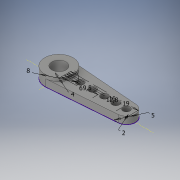
# Autodesk Inventor part: Servo-Arm-20mm
Saved by Autodesk Inventor 2018.2 (Build 222227000, 227)
## iProperties
Created: 2018-02-17
Part Number: Servo-Arm-20mm
Material: Generisch
Document SubType Name: Modeling
Designer: JochenAlt
Density: 1 g/cm^3
Appearance: Vorgabe
Author: JochenAlt
Autodesk Inventor part; units mm, degrees
ref_plane "YZ Plane" through (0, 0, 0) normal (1, 0, 0) x (0, 1, 0)
ref_plane "XZ Plane" through (0, 0, 0) normal (0, 1, 0) x (-1, 0, 0)
ref_plane "XY Plane" through (0, 0, 0) normal (0, 0, 1) x (1, 0, 0)
sketch "Skizze1" plane through (0, 0, 0) normal (0, 0, 1) x (1, 0, 0)
  line L0 (0, 5.6) -> (0, -5.6) construction
  line L1 (-9.1, 0) -> (26.6, 0) construction
  circle A0 centre (0, 0) radius 2
  circle A1 centre (9.5, 0) radius 1
  circle A2 centre (16, 0) radius 1
  circle A3 centre (19, 0) radius 1
  arc A4 (19.1974, -2.4922) -> (19.1974, 2.4922) centre (19, 0) ccw
  arc A5 (0.3158, 3.9875) -> (0.3158, -3.9875) centre (0, 0) ccw
  line L2 (0.3158, 3.9875) -> (19.1974, 2.4922)
  line L3 (0.3158, -3.9875) -> (19.1974, -2.4922)
  circle A6 centre (6, 0) radius 1
  circle A7 centre (12.8, 0) radius 1
  circle A8 centre (0, 0) radius 4
  point P0 (0.5263, 3.9652)
  point P1 (0.6579, -1.8887)
  point P2 (0.6579, 1.8887)
  dimension "d0" = 9.5
  dimension "d1" = 16
  dimension "d2" = 19
  dimension "d3" = 5
  dimension "d4" = 2
  dimension "d5" = 4
  dimension "d6" = 8
  dimension "d16" = 6
  dimension "d17" = 12.8
  constraints: 8 centre point, 7 point on circle, 5 point on line, 4 coincident, 4 end point, 4 equal radius, 4 tangent, 3 other
  measures "d0" distance of A1.centre point (0, 0)
  measures "d1" distance of point (0, 0) A2.centre
  measures "d2" distance of A3.centre point (0, 0)
  measures "d3" diameter of A4
  measures "d4" diameter of A3
  measures "d5" diameter of A0
  measures "d6" diameter of A5
  measures "d16" distance of A6.centre point (0, 0)
  measures "d17" distance of A7.centre point (0, 0)
extrude "Extrusion1" add sketch "Skizze1" along normal blind 2
extrude "Extrusion2" add sketch "Skizze1" along normal blind 3 contours A5 A8
